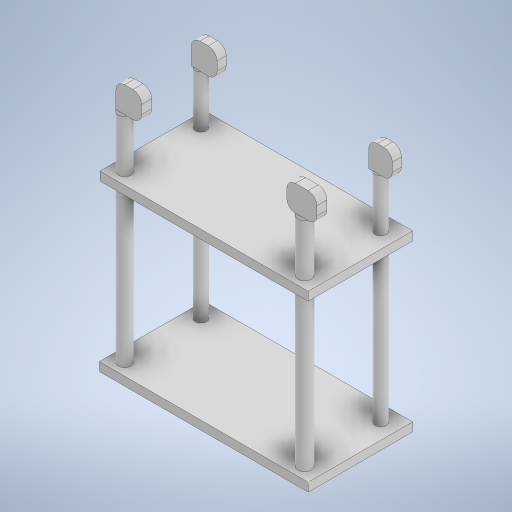
# Autodesk Inventor part: Rolling cart
Saved by Autodesk Inventor 2023.2 (Build 272271000, 271)
## iProperties
Created: 2022-12-08
Part Number: Rolling cart
Material: Generic
Document SubType Name: Modeling
Designer: Team 4026
Density: 1 g/cm^3
Appearance: Default
Author: Team 4026
Autodesk Inventor part; units mm, degrees
ref_plane "YZ Plane" through (0, 0, 0) normal (1, 0, 0) x (0, 1, 0)
ref_plane "XZ Plane" through (0, 0, 0) normal (0, 1, 0) x (-1, 0, 0)
ref_plane "XY Plane" through (0, 0, 0) normal (0, 0, 1) x (1, 0, 0)
sketch "Sketch1" plane through (0, 0, 0) normal (0, 1, 0) x (-1, 0, 0)
  line L0 (0, 0) -> (609.6, 0)
  line L1 (609.6, 0) -> (609.6, -304.8)
  line L2 (609.6, -304.8) -> (0, -304.8)
  line L3 (0, -304.8) -> (0, 0)
  dimension "d0" = 609.6
  dimension "d1" = 304.8
  constraints: 8 end point, 2 parallel, 1 horizontal, 1 perpendicular
  measures "d0" distance of L1.end L2.end
  measures "d1" distance of L0.end L1.end
extrude "Extrusion1" add sketch "Sketch1" along normal blind 25.4
sketch "Sketch2" plane through (0, 25.4, 0) normal (0, 1, 0) x (1, 0, 0)
  circle A0 centre (-570.3322, 34.6294) radius 18.7949
  circle A1 centre (-570.3322, 257.2374) radius 16.6125
  circle A2 centre (-45.3761, 34.6294) radius 19.935
  circle A3 centre (-45.3761, 257.2374) radius 16.6125
  point P0 (0, 0)
  constraints: 4 centre point
extrude "Extrusion3" add sketch "Sketch2" along normal blind 457.2
sketch "Sketch3" plane through (-570.3322, 482.6, -34.6294) normal (0, 1, 0) x (1, 0, 0)
  line L0 (-37.29, -34.6294) -> (570.3322, -34.6294)
  line L1 (570.3322, -34.6294) -> (570.3322, 270.1706)
  line L2 (570.3322, 270.1706) -> (-37.29, 270.1706)
  line L3 (-37.29, 270.1706) -> (-37.29, -34.6294)
  constraints: 8 end point, 2 parallel, 1 horizontal, 1 perpendicular
extrude "Extrusion4" add sketch "Sketch3" along normal blind 25.4
sketch "Sketch4" plane through (0, 25.4, 0) normal (0, 1, 0) x (1, 0, 0)
  point P0 (0, 0)
sketch "Sketch6" plane through (-570.3322, 508, -34.6294) normal (0, 1, 0) x (1, 0, 0)
  circle A0 centre (0, 222.608) radius 16.6125 projected
  circle A1 centre (0, 222.608) radius 23.4937
  circle A2 centre (524.9562, 222.608) radius 16.6125 projected
  circle A3 centre (524.9562, 222.608) radius 21.1362
  circle A4 centre (524.9562, 0) radius 19.935 projected
  circle A5 centre (524.9562, 0) radius 19.935
  circle A6 centre (0, 0) radius 18.7949 projected
  circle A7 centre (0, 0) radius 18.7949
  point P0 (570.3322, -34.6294)
  constraints: 4 centre point, 4 coincident
extrude "Extrusion5" add sketch "Sketch6" along normal blind 152.4 contours A0 | A2 | A4 | A6
sketch "Sketch7" plane through (-570.3322, 660.4, -34.6294) normal (0, 1, 0) x (1, 0, 0)
  circle A0 centre (0, 0) radius 18.7949 projected
  line L0 (-16.3638, -9.2453) -> (58.6453, -9.2453)
  line L1 (58.6453, -9.2453) -> (58.6453, 20.1685)
  line L2 (58.6453, 20.1685) -> (-16.3638, 20.1685)
  line L3 (-16.3638, 20.1685) -> (-16.3638, -9.2453)
  line L4 (-16.3638, 210.9623) -> (58.6453, 210.9623)
  line L5 (58.6453, 210.9623) -> (58.6453, 237.7194)
  line L6 (58.6453, 237.7194) -> (-16.3638, 237.7194)
  line L7 (-16.3638, 237.7194) -> (-16.3638, 210.9623)
  line L8 (482.4161, -9.2453) -> (570.3322, -9.2453)
  line L9 (570.3322, -9.2453) -> (570.3322, 20.1685)
  line L10 (570.3322, 20.1685) -> (482.4161, 20.1685)
  line L11 (482.4161, 20.1685) -> (482.4161, -9.2453)
  line L12 (570.3322, -34.6294) -> (570.3322, 270.1706) projected
  line L13 (501.5283, 210.9623) -> (570.3322, 210.9623)
  line L14 (570.3322, 210.9623) -> (570.3322, 237.7194)
  line L15 (570.3322, 237.7194) -> (501.5283, 237.7194)
  line L16 (501.5283, 237.7194) -> (501.5283, 210.9623)
  constraints: 32 end point, 8 parallel, 7 point on line, 4 horizontal, 4 perpendicular, 2 other
extrude "Extrusion6" add sketch "Sketch7" along normal blind 76.2 contours A0 L0 L3 | A0 L3 L2 L1 L0 | L7 L6 L5 L4 | L11 L10 L9 L8 | L13 L16 L15 L12
fillet "Fillet1" radius 25.4 1 edges at (0, 736.6, -40.091)
fillet "Fillet2" radius 25.4 9 edges at (-586.6961, 736.6, -258.9703) (-511.687, 736.6, -258.9703) (-586.6961, 736.6, -40.091) (-511.687, 736.6, -40.091) (-87.9161, 736.6, -40.091) (-68.8039, 736.6, -258.9703) (0, 736.6, -258.9703) (-87.9161, 660.4, -40.091) (-511.687, 660.4, -40.091)
fillet "Fillet3" radius 25.4 3 edges at (0, 660.4, -258.9703) (-511.687, 660.4, -258.9703) (0, 660.4, -40.091)
body "Solid1"
